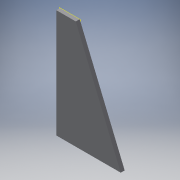
# Autodesk Inventor part: internalSupportBottom3
Saved by Autodesk Inventor 2019 (Build 230136000, 136)
## iProperties
Created: 2019-01-08
Part Number: internalSupportBottom3
Material: Wood (Birch)
Document SubType Name: Modeling
Designer: gaincarlo
Density: 0.55 g/cm^3
Appearance: Birch - Natural Polished
Author: gaincarlo
Autodesk Inventor part; units mm, degrees
ref_plane "YZ Plane" through (0, 0, 0) normal (1, 0, 0) x (0, 1, 0)
ref_plane "XZ Plane" through (0, 0, 0) normal (0, 1, 0) x (-1, 0, 0)
ref_plane "Work Plane1" through (0, 0, 0) normal (0, 0, 1) x (1, 0, 0)
sketch "Sketch1" plane through (0, 0, 0) normal (0, 0, 1) x (1, 0, 0)
  line L0 (-50, 3) -> (0, 3) construction
  spline S0 degree 3 poles (2.7714, 4.1486) (21.9049, -42.0198) (41.3, -88.8125) (79.5731, -181.141) (98.9279, -227.827) (118.0713, -274) knots -29.96646 -29.96646 -29.96646 -29.96646 -14.995258 -14.995258 0 0 0 0 construction
  spline S1 degree 3 poles (118.0713, -274) (117.6094, -274.1915) (117.1476, -274.383) (116.2238, -274.766) (115.7619, -274.9574) (115.3, -275.1489) knots -0.30001 -0.30001 -0.30001 -0.30001 -0.150005 -0.150005 0 0 0 0 construction
  spline S2 degree 3 poles (115.3, -275.1489) (96.1483, -228.9562) (76.787, -182.2543) (38.5123, -89.9219) (19.1268, -43.1522) (0, 3) knots -30.011396 -30.011396 -30.011396 -30.011396 -14.988387 -14.988387 -0.000837 -0.000837 -0.000837 -0.000837 construction
  spline S3 degree 3 poles (0, 3) (0.4619, 3.1914) (0.9238, 3.3829) (1.8476, 3.7657) (2.3095, 3.9571) (2.7714, 4.1486) knots -0.3 -0.3 -0.3 -0.3 -0.15 -0.15 0 0 0 0 construction
  line L1 (0, 3) -> (-50, 3)
  line L2 (-50, -275.1489) -> (115.3, -275.1489)
  line L3 (0, 3) -> (115.3, -275.1489)
  line L4 (-50, 3) -> (-50, -275.1489)
  point P0 (0, 0)
  constraints: 8 end point, 2 perpendicular, 1 horizontal, 15 other
extrude "Extrusion1" add sketch "Sketch1" along normal blind 10
body "Solid1"
